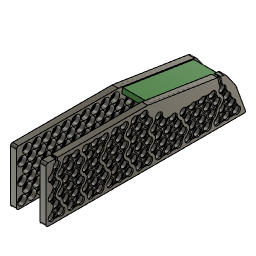
battery v13 (Autodesk Fusion 360 design; units mm, degrees)
Autodesk Fusion 360 part; units mm, degrees
note: some values were not read from the file. Set by a fixed rule: which face or edge a step refers to.
(part 1 of 2)
sketch "Sketch1" plane through (0, 0, 0) normal (1, 0, 0) x (0, 1, 0)
  circle A0 centre (0, 0) radius 9.25
  circle A1 centre (19.5, 0) radius 9.25
  circle A2 centre (39, 0) radius 9.25
  circle A3 centre (58.5, 0) radius 9.25
  circle A4 centre (78, 0) radius 9.25
  circle A5 centre (97.5, 0) radius 9.25
  circle A6 centre (117, 0) radius 9.25
  circle A7 centre (136.5, 0) radius 9.25
  circle A8 centre (156, 0) radius 9.25
  circle A9 centre (175.5, 0) radius 9.25
  circle A10 centre (195, 0) radius 9.25
  circle A11 centre (214.5, 0) radius 9.25
  circle A12 centre (234, 0) radius 9.25
  circle A13 centre (253.5, 0) radius 9.25
  circle A14 centre (273, 0) radius 9.25
  circle A15 centre (292.5, 0) radius 9.25
  circle A16 centre (312, 0) radius 9.25
  circle A17 centre (331.5, 0) radius 9.25
  circle A18 centre (351, 0) radius 9.25
  circle A19 centre (127, 17) radius 9.25
  circle A20 centre (88, 17) radius 9.25
  circle A21 centre (283, 17) radius 9.25
  circle A22 centre (263.5, 17) radius 9.25
  circle A23 centre (10, 17) radius 9.25
  circle A24 centre (68.5, 17) radius 9.25
  circle A25 centre (185.5, 17) radius 9.25
  circle A26 centre (205, 17) radius 9.25
  circle A27 centre (107.5, 17) radius 9.25
  circle A28 centre (166, 17) radius 9.25
  circle A29 centre (-9.5, 17) radius 9.25
  circle A30 centre (302.5, 17) radius 9.25
  circle A31 centre (146.5, 17) radius 9.25
  circle A32 centre (224.5, 17) radius 9.25
  circle A33 centre (49, 17) radius 9.25
  circle A34 centre (341.5, 17) radius 9.25
  circle A35 centre (322, 17) radius 9.25
  circle A36 centre (244, 17) radius 9.25
  circle A37 centre (29.5, 17) radius 9.25
  circle A38 centre (58.5, 34) radius 9.25
  circle A39 centre (214.5, 34) radius 9.25
  circle A40 centre (136.5, 34) radius 9.25
  circle A41 centre (19.5, 34) radius 9.25
  circle A42 centre (195, 34) radius 9.25
  circle A43 centre (78, 34) radius 9.25
  circle A44 centre (175.5, 34) radius 9.25
  circle A45 centre (253.5, 34) radius 9.25
  circle A46 centre (331.5, 34) radius 9.25
  circle A47 centre (0, 34) radius 9.25
  circle A48 centre (234, 34) radius 9.25
  circle A49 centre (39, 34) radius 9.25
  circle A50 centre (156, 34) radius 9.25
  circle A51 centre (97.5, 34) radius 9.25
  circle A52 centre (117, 34) radius 9.25
  circle A53 centre (292.5, 34) radius 9.25
  circle A54 centre (312, 34) radius 9.25
  circle A55 centre (273, 34) radius 9.25
  circle A56 centre (185.4697, 51) radius 9.25
  circle A57 centre (263.4697, 51) radius 9.25
  circle A58 centre (321.9697, 51) radius 9.25
  circle A59 centre (224.4697, 51) radius 9.25
  circle A60 centre (9.9697, 51) radius 9.25
  circle A61 centre (243.9697, 51) radius 9.25
  circle A62 centre (282.9697, 51) radius 9.25
  circle A63 centre (302.4697, 51) radius 9.25
  circle A64 centre (48.9697, 51) radius 9.25
  circle A65 centre (29.4697, 51) radius 9.25
  circle A66 centre (-9.5303, 51) radius 9.25
  circle A67 centre (107.4697, 51) radius 9.25
  circle A68 centre (165.9697, 51) radius 9.25
  circle A69 centre (204.9697, 51) radius 9.25
  circle A70 centre (87.9697, 51) radius 9.25
  circle A71 centre (68.4697, 51) radius 9.25
  circle A72 centre (146.4697, 51) radius 9.25
  circle A73 centre (126.9697, 51) radius 9.25
  circle A74 centre (-19.5, 34) radius 9.25
  circle A75 centre (-19.5, 0) radius 9.25
  circle A76 centre (351, 0) radius 7
  circle A77 centre (331.5, 0) radius 7
  circle A78 centre (312, 0) radius 7
  circle A79 centre (292.5, 0) radius 7
  circle A80 centre (273, 0) radius 7
  circle A81 centre (253.5, 0) radius 7
  circle A82 centre (234, 0) radius 7
  circle A83 centre (214.5, 0) radius 7
  circle A84 centre (195, 0) radius 7
  circle A85 centre (175.5, 0) radius 7
  circle A86 centre (156, 0) radius 7
  circle A87 centre (136.5, 0) radius 7
  circle A88 centre (117, 0) radius 7
  circle A89 centre (97.5, 0) radius 7
  circle A90 centre (78, 0) radius 7
  circle A91 centre (58.5, 0) radius 7
  circle A92 centre (39, 0) radius 7
  circle A93 centre (19.5, 0) radius 7
  circle A94 centre (0, 0) radius 7
  circle A95 centre (-19.5, 0) radius 7
  circle A96 centre (341.5, 17) radius 7
  circle A97 centre (331.5, 34) radius 7
  circle A98 centre (321.9697, 51) radius 7
  circle A99 centre (322, 17) radius 7
  circle A100 centre (312, 34) radius 7
  circle A101 centre (302.4697, 51) radius 7
  circle A102 centre (302.5, 17) radius 7
  circle A103 centre (292.5, 34) radius 7
  circle A104 centre (282.9697, 51) radius 7
  circle A105 centre (283, 17) radius 7
  circle A106 centre (273, 34) radius 7
  circle A107 centre (263.4697, 51) radius 7
  circle A108 centre (263.5, 17) radius 7
  circle A109 centre (253.5, 34) radius 7
  circle A110 centre (243.9697, 51) radius 7
  circle A111 centre (244, 17) radius 7
  circle A112 centre (234, 34) radius 7
  circle A113 centre (224.4697, 51) radius 7
  circle A114 centre (224.5, 17) radius 7
  circle A115 centre (214.5, 34) radius 7
  circle A116 centre (204.9697, 51) radius 7
  circle A117 centre (205, 17) radius 7
  circle A118 centre (195, 34) radius 7
  circle A119 centre (185.4697, 51) radius 7
  circle A120 centre (185.5, 17) radius 7
  circle A121 centre (175.5, 34) radius 7
  circle A122 centre (165.9697, 51) radius 7
  circle A123 centre (166, 17) radius 7
  circle A124 centre (156, 34) radius 7
  circle A125 centre (146.4697, 51) radius 7
  circle A126 centre (146.5, 17) radius 7
  circle A127 centre (136.5, 34) radius 7
  circle A128 centre (126.9697, 51) radius 7
  circle A129 centre (127, 17) radius 7
  circle A130 centre (117, 34) radius 7
  circle A131 centre (107.4697, 51) radius 7
  circle A132 centre (107.5, 17) radius 7
  circle A133 centre (97.5, 34) radius 7
  circle A134 centre (87.9697, 51) radius 7
  circle A135 centre (88, 17) radius 7
  circle A136 centre (78, 34) radius 7
  circle A137 centre (68.4697, 51) radius 7
  circle A138 centre (68.5, 17) radius 7
  circle A139 centre (58.5, 34) radius 7
  circle A140 centre (48.9697, 51) radius 7
  circle A141 centre (49, 17) radius 7
  circle A142 centre (39, 34) radius 7
  circle A143 centre (29.4697, 51) radius 7
  circle A144 centre (29.5, 17) radius 7
  circle A145 centre (19.5, 34) radius 7
  circle A146 centre (9.9697, 51) radius 7
  circle A147 centre (10, 17) radius 7
  circle A148 centre (0, 34) radius 7
  circle A149 centre (-9.5303, 51) radius 7
  circle A150 centre (-9.5, 17) radius 7
  circle A151 centre (-19.5, 34) radius 7
  line L0 (-31, -12) -> (-31, 98)
  line L1 (-31, -12) -> (369, -12)
  line L2 (-31, 98) -> (172.6327, 98)
  line L3 (327.7275, 73.6318) -> (348.4062, 44.7862)
  line L4 (348.4062, 44.7862) -> (369, -12)
  line L5 (172.6327, 98) -> (327.7275, 73.6318)
  circle A152 centre (-19.5, 68) radius 9.25
  circle A153 centre (-19.5, 68) radius 7
  circle A154 centre (-9.5303, 85) radius 9.25
  circle A155 centre (-9.5303, 85) radius 7
  circle A156 centre (0, 68) radius 9.25
  circle A157 centre (0, 68) radius 7
  circle A158 centre (9.9697, 85) radius 9.25
  circle A159 centre (9.9697, 85) radius 7
  circle A160 centre (19.5, 68) radius 9.25
  circle A161 centre (19.5, 68) radius 7
  circle A162 centre (29.4697, 85) radius 9.25
  circle A163 centre (29.4697, 85) radius 7
  circle A164 centre (39, 68) radius 9.25
  circle A165 centre (39, 68) radius 7
  circle A166 centre (48.9697, 85) radius 9.25
  circle A167 centre (48.9697, 85) radius 7
  circle A168 centre (58.5, 68) radius 9.25
  circle A169 centre (58.5, 68) radius 7
  circle A170 centre (68.4697, 85) radius 9.25
  circle A171 centre (68.4697, 85) radius 7
  circle A172 centre (78, 68) radius 9.25
  circle A173 centre (78, 68) radius 7
  circle A174 centre (87.9697, 85) radius 9.25
  circle A175 centre (87.9697, 85) radius 7
  circle A176 centre (97.5, 68) radius 9.25
  circle A177 centre (97.5, 68) radius 7
  circle A178 centre (107.4697, 85) radius 9.25
  circle A179 centre (107.4697, 85) radius 7
  circle A180 centre (117, 68) radius 9.25
  circle A181 centre (117, 68) radius 7
  circle A182 centre (126.9697, 85) radius 9.25
  circle A183 centre (126.9697, 85) radius 7
  circle A184 centre (136.5, 68) radius 9.25
  circle A185 centre (136.5, 68) radius 7
  circle A186 centre (146.4697, 85) radius 9.25
  circle A187 centre (146.4697, 85) radius 7
  circle A188 centre (156, 68) radius 9.25
  circle A189 centre (156, 68) radius 7
  circle A190 centre (165.9697, 85) radius 9.25
  circle A191 centre (165.9697, 85) radius 7
  circle A192 centre (175.5, 68) radius 9.25
  circle A193 centre (175.5, 68) radius 7
  circle A194 centre (195, 68) radius 7
  circle A195 centre (195, 68) radius 9.25
  point P0 (-9.5, 17)
  point P1 (0, 34)
  point P2 (-9.5303, 51)
  dimension "d4" = 19.5
  dimension "d5" = 0
  dimension "d8" = 19.5
  dimension "d9" = 0
  dimension "d13" = 19.5
  dimension "d14" = 0
  dimension "d18" = 19.5
  dimension "d19" = 0
  dimension "d28" = 14
  dimension "d31" = -19.5
  dimension "d32" = 0
  dimension "d33" = 14
  dimension "d34" = 14
  dimension "d35" = 14
  dimension "d40" = -19.5
  dimension "d41" = 0
  dimension "d48" = 12
  dimension "d252" = 18.5
  dimension "d253" = 18.5
  dimension "d254" = 17
  dimension "d255" = 17
  dimension "d256" = 18.5
  dimension "d257" = 19.5
  dimension "d258" = 18.5
  dimension "d259" = 18.5
  dimension "d260" = 17
  dimension "d262" = 18.5
  dimension "d265" = 17
  dimension "d268" = 400
  dimension "d271" = 19.5
  dimension "d272" = 34
  dimension "d273" = 110
  dimension "d276" = 19.5
  dimension "d277" = 19.5
  constraint coincident A0.centre A94.centre
  constraint coincident P0 A29.centre
  constraint coincident P1 A47.centre
  constraint coincident P2 A66.centre
  constraint concentric A18 A76
  constraint concentric A34 A96
  constraint concentric A46 A97
  constraint concentric A58 A98
  constraint vertical L0
  constraint horizontal L1
  constraint horizontal L2
  constraint coincident A75.centre A95.centre
  constraint coincident A74.centre A151.centre
  measures "d28" diameter of A76
  measures "d33" diameter of A96
  measures "d34" diameter of A97
  measures "d35" diameter of A98
  measures "d48" distance of A75.centre L1
  measures "d252" diameter of A0
  measures "d253" diameter of A34
  measures "d254" vertical distance of A18.centre A34.centre
  measures "d255" vertical distance of A46.centre A34.centre
  measures "d256" diameter of A75
  measures "d257" horizontal distance of P1 A74.centre
  measures "d258" diameter of A74
  measures "d259" diameter of A47
  measures "d260" vertical distance of P1 P2
  measures "d262" diameter of A58
  measures "d265" vertical distance of P0 A74.centre
  measures "d268" distance of L0.start L1.end
  measures "d273" distance of L0.end L0.start
extrude "Extrude1" add sketch "Sketch1" along normal blind 12 contours L0 L1 L2 L3 L4 L5 makes body 1
extrude "Extrude2" add sketch "Sketch1" along normal blind 3 contours A0 | A1 | A2 | A3 | A4 | A5 | A6 | A7 | A8 | A9 | A10 | A11 | A12 | A13 | A14 | A15 | A16 | A17 | A18 | A19 | A20 | A21 | A22 | A23 | A24 | A25 | A26 | A27 | A28 | A29 | A30 | A31 | A32 | A33 | A34 | A35 | A36 | A37 | A38 | A39 | A40 | A41 | A42 | A43 | A44 | A45 | A46 | A47 | A48 | A49 | A50 | A51 | A52 | A53 | A54 | A55 | A56 | A57 | A58 | A59 | A60 | A61 | A62 | A63 | A64 | A65 | A66 | A67 | A68 | A69 | A70 | A71 | A72 | A73 | A74 | A75 | A152 | A154 | A156 | A158 | A160 | A162 | A164 | A166 | A168 | A170 | A172 | A174 | A176 | A178 | A180 | A182 | A184 | A186 | A188 | A190 | A192 | A195 bodies 1
sketch "Sketch2" plane through (0, 0, 0) normal (-1, 0, 0) x (0, -1, 0)
  circle A0 centre (-331.5, 0) radius 7 construction
  circle A1 centre (-322, 17) radius 7 construction
  circle A2 centre (-312, 34) radius 7 construction
  circle A3 centre (-283, 17) radius 7 construction
  circle A4 centre (-273, 34) radius 7 construction
  circle A5 centre (-244, 17) radius 7 construction
  circle A6 centre (-224.5, 17) radius 7 construction
  circle A7 centre (-214.5, 34) radius 7 construction
  circle A8 centre (-185.5, 17) radius 7 construction
  circle A9 centre (-117, 0) radius 7 construction
  circle A10 centre (-146.5, 17) radius 7 construction
  circle A11 centre (-165.9697, 51) radius 7 construction
  circle A12 centre (-117, 34) radius 7 construction
  circle A13 centre (-88, 17) radius 7 construction
  circle A14 centre (-68.5, 17) radius 7 construction
  circle A15 centre (-39, 34) radius 7 construction
  circle A16 centre (-29.4697, 51) radius 7 construction
  circle A17 centre (-9.9697, 51) radius 7 construction
  circle A18 centre (0, 0) radius 7 construction
  circle A19 centre (9.5, 17) radius 7 construction
  circle A20 centre (19.5, 34) radius 7 construction
  circle A21 centre (9.5303, 51) radius 7 construction
  circle A22 centre (-19.5, 0) radius 7 construction
  circle A23 centre (-49, 17) radius 7 construction
  circle A24 centre (-78, 34) radius 7 construction
  circle A25 centre (-78, 0) radius 7 construction
  circle A26 centre (-126.9697, 51) radius 7 construction
  circle A27 centre (-185.4697, 51) radius 7 construction
  circle A28 centre (-136.5, 34) radius 7 construction
  circle A29 centre (-156, 0) radius 7 construction
  circle A30 centre (-195, 34) radius 7 construction
  circle A31 centre (-205, 17) radius 7 construction
  circle A32 centre (-234, 34) radius 7 construction
  circle A33 centre (-253.5, 34) radius 7 construction
  circle A34 centre (-263.5, 17) radius 7 construction
  circle A35 centre (-292.5, 34) radius 7 construction
  circle A36 centre (-302.5, 17) radius 7 construction
  circle A37 centre (-331.5, 34) radius 7 construction
  circle A38 centre (-351, 0) radius 7 construction
  circle A39 centre (-312, 0) radius 7 construction
  circle A40 centre (-321.9697, 51) radius 7 construction
  circle A41 centre (-273, 0) radius 7 construction
  circle A42 centre (-282.9697, 51) radius 7 construction
  circle A43 centre (-234, 0) radius 7 construction
  circle A44 centre (-214.5, 0) radius 7 construction
  circle A45 centre (-224.4697, 51) radius 7 construction
  circle A46 centre (-175.5, 0) radius 7 construction
  circle A47 centre (-136.5, 0) radius 7 construction
  circle A48 centre (-156, 34) radius 7 construction
  circle A49 centre (-146.4697, 51) radius 7 construction
  circle A50 centre (-107.5, 17) radius 7 construction
  circle A51 centre (-97.5, 34) radius 7 construction
  circle A52 centre (-58.5, 0) radius 7 construction
  circle A53 centre (-58.5, 34) radius 7 construction
  circle A54 centre (-19.5, 34) radius 7 construction
  circle A55 centre (-10, 17) radius 7 construction
  circle A56 centre (19.5, 0) radius 7 construction
  circle A57 centre (0, 34) radius 7 construction
  circle A58 centre (-29.5, 17) radius 7 construction
  circle A59 centre (-48.9697, 51) radius 7 construction
  circle A60 centre (-39, 0) radius 7 construction
  circle A61 centre (-68.4697, 51) radius 7 construction
  circle A62 centre (-87.9697, 51) radius 7 construction
  circle A63 centre (-97.5, 0) radius 7 construction
  circle A64 centre (-107.4697, 51) radius 7 construction
  circle A65 centre (-175.5, 34) radius 7 construction
  circle A66 centre (-127, 17) radius 7 construction
  circle A67 centre (-166, 17) radius 7 construction
  circle A68 centre (-204.9697, 51) radius 7 construction
  circle A69 centre (-195, 0) radius 7 construction
  circle A70 centre (-243.9697, 51) radius 7 construction
  circle A71 centre (-263.4697, 51) radius 7 construction
  circle A72 centre (-253.5, 0) radius 7 construction
  circle A73 centre (-302.4697, 51) radius 7 construction
  circle A74 centre (-292.5, 0) radius 7 construction
  circle A75 centre (-341.5, 17) radius 7 construction
  line L0 (-327.7275, 73.6318) -> (-348.4062, 44.7862) construction
  line L1 (-348.4062, 44.7862) -> (-369, -12) construction
  line L2 (-369, -12) -> (31, -12)
  line L3 (31, -12) -> (31, 98)
  line L4 (31, 98) -> (-172.6327, 98)
  line L5 (9.5303, 85) -> (19.4283, 67.8265) construction
  line L6 (19.4283, 67.8265) -> (9.5303, 51) construction
  line L7 (9.5303, 51) -> (19.5, 34) construction
  line L8 (19.5, 34) -> (9.5, 17) construction
  line L9 (0, 0) -> (9.5, 17) construction
  line L10 (-19.5, 0) -> (-10, 17) construction
  line L11 (-10, 17) -> (0, 34) construction
  line L12 (0, 34) -> (-9.9697, 51) construction
  line L13 (-9.9697, 51) -> (0, 68) construction
  line L14 (0, 68) -> (-9.9697, 85) construction
  line L15 (-9.9697, 85) -> (-19.5, 68) construction
  line L16 (-19.5, 68) -> (-9.9697, 51) construction
  line L17 (-39, 0) -> (-29.5, 17) construction
  line L18 (-29.5, 17) -> (-19.5, 34) construction
  line L19 (-19.5, 34) -> (-29.4697, 51) construction
  line L20 (-29.4697, 51) -> (-39, 68) construction
  line L21 (-39, 68) -> (-29.4697, 85) construction
  line L22 (-39, 34) -> (-29.5, 17) construction
  line L23 (-39, 34) -> (-29.4697, 51) construction
  line L24 (-58.5, 0) -> (-49, 17) construction
  line L25 (-49, 17) -> (-58.5, 34) construction
  line L26 (-58.5, 34) -> (-48.9697, 51) construction
  line L27 (-48.9697, 51) -> (-58.5, 68) construction
  line L28 (-58.5, 68) -> (-48.9697, 85) construction
  line L29 (-48.9697, 85) -> (-68.4697, 85) construction
  line L30 (-68.4697, 85) -> (-58.5, 68) construction
  line L31 (-78, 0) -> (-68.5, 17) construction
  line L32 (-68.5, 17) -> (-78, 34) construction
  line L33 (-78, 34) -> (-68.4697, 51) construction
  line L34 (-68.4697, 51) -> (-76.7499, 65.5682) construction
  line L35 (-76.7499, 65.5682) -> (-87.9697, 85) construction
  line L36 (-78, 0) -> (-88, 17) construction
  line L37 (-88, 17) -> (-78, 34) construction
  line L38 (-97.5, 0) -> (-107.5, 17) construction
  line L39 (-107.5, 17) -> (-97.5, 34) construction
  line L40 (-97.5, 34) -> (-87.9697, 51) construction
  line L41 (-87.9697, 51) -> (-97.5, 68) construction
  line L42 (-97.5, 68) -> (-107.4697, 51) construction
  line L43 (-107.4697, 51) -> (-97.5, 34) construction
  line L44 (-97.5, 68) -> (-107.4697, 85) construction
  line L45 (-126.9697, 85) -> (-117, 68) construction
  line L46 (-117, 68) -> (-126.9697, 51) construction
  line L47 (-126.9697, 51) -> (-117, 34) construction
  line L48 (-117, 34) -> (-127, 17) construction
  line L49 (-127, 17) -> (-117, 0) construction
  line L50 (-117, 0) -> (-136.5, 0) construction
  line L51 (-136.5, 0) -> (-127, 17) construction
  line L52 (-156, 0) -> (-146.5, 17) construction
  line L53 (-146.5, 17) -> (-136.5, 34) construction
  line L54 (-136.5, 34) -> (-146.4697, 51) construction
  line L55 (-146.4697, 51) -> (-136.5, 68) construction
  line L56 (-136.5, 68) -> (-146.4697, 85) construction
  line L57 (-156, 34) -> (-146.5, 17) construction
  line L58 (-156, 34) -> (-146.4697, 51) construction
  line L59 (-165.9697, 85) -> (-156, 68) construction
  line L60 (-175.5, 68) -> (-165.9697, 85) construction
  line L61 (-165.9697, 51) -> (-156, 68) construction
  line L62 (-165.9697, 51) -> (-175.5, 34) construction
  line L63 (-175.5, 34) -> (-166, 17) construction
  line L64 (-166, 17) -> (-175.5, 0) construction
  line L65 (-175.5, 68) -> (-165.9697, 51) construction
  line L66 (-195, 0) -> (-185.5, 17) construction
  line L67 (-185.5, 17) -> (-195, 34) construction
  line L68 (-195, 34) -> (-185.4697, 51) construction
  line L69 (-185.4697, 51) -> (-195, 68) construction
  line L70 (-204.9697, 51) -> (-195, 34) construction
  line L71 (-195, 68) -> (-204.9697, 51) construction
  line L72 (-205, 17) -> (-195, 0) construction
  line L73 (-205, 17) -> (-195, 34) construction
  line L74 (-214.5, 34) -> (-224.4697, 51) construction
  line L75 (-224.4697, 51) -> (-234, 34) construction
  line L76 (-224.5, 17) -> (-214.5, 0) construction
  line L77 (-214.5, 0) -> (-234, 0) construction
  line L78 (-224.5, 17) -> (-214.5, 34) construction
  line L79 (-234, 0) -> (-244, 17) construction
  line L80 (-244, 17) -> (-234, 34) construction
  line L81 (-243.9697, 51) -> (-263.4697, 51) construction
  line L82 (-253.5, 34) -> (-243.9697, 51) construction
  line L83 (-253.5, 34) -> (-263.5, 17) construction
  line L84 (-263.5, 17) -> (-253.5, 0) construction
  line L85 (-253.5, 0) -> (-273, 0) construction
  line L86 (-273, 0) -> (-263.5, 17) construction
  line L87 (-263.5, 17) -> (-273, 34) construction
  line L88 (-273, 34) -> (-263.4697, 51) construction
  line L89 (-282.9697, 51) -> (-292.5, 34) construction
  line L90 (-292.5, 34) -> (-283, 17) construction
  line L91 (-283, 17) -> (-292.5, 0) construction
  line L92 (-292.5, 0) -> (-302.5, 17) construction
  line L93 (-302.5, 17) -> (-312, 34) construction
  line L94 (-312, 34) -> (-302.4697, 51) construction
  line L95 (-351, 0) -> (-341.5, 17) construction
  line L96 (-341.5, 17) -> (-331.5, 34) construction
  line L97 (-331.5, 34) -> (-322, 17) construction
  line L98 (-351, 0) -> (-331.5, 0) construction
  line L99 (-312, 0) -> (-322, 17) construction
  line L100 (-331.5, 0) -> (-312, 0) construction
  line L101 (-321.9697, 51) -> (-331.5, 34) construction
  line L102 (-302.4697, 51) -> (-282.9697, 51) construction
  line L103 (-172.6327, 98) -> (-327.7275, 73.6318) construction
  circle A76 centre (-175.5, 68) radius 7 construction
  circle A77 centre (-146.4697, 85) radius 7 construction
  circle A78 centre (-107.4697, 85) radius 7 construction
  circle A79 centre (-68.4697, 85) radius 7 construction
  circle A80 centre (-29.4697, 85) radius 7 construction
  circle A81 centre (9.5303, 85) radius 7 construction
  circle A82 centre (-9.9697, 85) radius 7 construction
  circle A83 centre (-39, 68) radius 7 construction
  circle A84 centre (-78, 68) radius 7 construction
  circle A85 centre (-126.9697, 85) radius 7 construction
  circle A86 centre (-156, 68) radius 7 construction
  circle A87 centre (-136.5, 68) radius 7 construction
  circle A88 centre (-97.5, 68) radius 7 construction
  circle A89 centre (-58.5, 68) radius 7 construction
  circle A90 centre (-19.5, 68) radius 7 construction
  circle A91 centre (19.5, 68) radius 7 construction
  circle A92 centre (0, 68) radius 7 construction
  circle A93 centre (-48.9697, 85) radius 7 construction
  circle A94 centre (-87.9697, 85) radius 7 construction
  circle A95 centre (-117, 68) radius 7 construction
  circle A96 centre (-165.9697, 85) radius 7 construction
  circle A97 centre (-195, 68) radius 7 construction
  line L104 (-58.5977, 78.0505) -> (-57.5048, 80) construction
  line L105 (-57.5048, 80) -> (-59.741, 80) construction
  line L106 (-59.741, 80) -> (-58.5977, 78.0505) construction
  line L107 (-331.5, 0) -> (-322, 17) construction
  line L108 (-341.5, 17) -> (-331.5, 0) construction
  line L109 (-322, 17) -> (-341.5, 17) construction
  line L110 (-302.5, 17) -> (-283, 17) construction
  line L111 (-292.5, 34) -> (-312, 34) construction
  line L112 (-292.5, 34) -> (-302.5, 17) construction
  line L113 (-292.5, 34) -> (-302.4697, 51) construction
  line L114 (-253.5, 34) -> (-263.4697, 51) construction
  line L115 (-273, 34) -> (-253.5, 34) construction
  line L116 (-244, 17) -> (-224.5, 17) construction
  line L117 (-234, 0) -> (-224.5, 17) construction
  line L118 (-224.5, 17) -> (-234, 34) construction
  line L119 (-214.5, 34) -> (-234, 34) construction
  line L120 (-185.5, 17) -> (-205, 17) construction
  line L121 (-185.4697, 51) -> (-204.9697, 51) construction
  line L122 (-175.5, 68) -> (-156, 68) construction
  line L123 (-156, 34) -> (-136.5, 34) construction
  line L124 (-107.4697, 51) -> (-87.9697, 51) construction
  line L125 (-88, 17) -> (-68.5, 17) construction
  line L126 (-39, 34) -> (-19.5, 34) construction
  line L127 (-19.5, 68) -> (0, 68) construction
  line L128 (19.5, 0) -> (9.5, 17) construction
  line L129 (0, 0) -> (19.5, 0) construction
  line L130 (-335.5965, 16.8256) -> (-329.3321, 6.1762)
  line L131 (-344.2941, 12) -> (-344.3597, 12)
  line L132 (-344.3597, 12) -> (-337.7357, 0.7392)
  line L133 (-335.5965, 16.8256) -> (-337.4264, 19.9364)
  line L134 (-344.3597, 12) -> (-346.7144, 16.0029)
  line L135 (-337.7357, 0.7392) -> (-335.7099, -2.7047)
  line L136 (-329.3321, 6.1762) -> (-326.75, 1.781)
  line L137 (-335.7099, -2.7047) -> (-326.75, 1.781)
  line L138 (-337.4264, 19.9364) -> (-346.7144, 16.0029)
  line L139 (5.1983, 82.5033) -> (15.0963, 65.3298)
  line L140 (13.8623, 87.4967) -> (23.7603, 70.3233)
  line L141 (23.7603, 70.3233) -> (74.0347, -16.9057)
  line L142 (15.0963, 65.3298) -> (63.6851, -18.9746)
  line L143 (15.1903, 36.5351) -> (5.1903, 19.5351)
  line L144 (23.8097, 31.4649) -> (13.8097, 14.4649)
  line L145 (23.8097, 31.4649) -> (58.8391, 91.015)
  line L146 (15.1903, 36.5351) -> (49.1846, 94.3253)
  line L147 (5.1903, 19.5351) -> (-25, -30)
  line L148 (13.8097, 14.4649) -> (-15, -35)
  line L149 (5.1983, 82.5033) -> (0.3906, 90.845)
  line L150 (-5.6377, 87.4967) -> (4.2603, 70.3233)
  line L151 (4.2603, 70.3233) -> (54.5347, -16.9057)
  line L152 (-14.3017, 82.5033) -> (-19.1094, 90.845)
  line L153 (-14.3017, 82.5033) -> (-4.4037, 65.3298)
  line L154 (-4.4037, 65.3298) -> (44.1851, -18.9746)
  line L155 (-25.1377, 87.4967) -> (-15.2397, 70.3233)
  line L156 (-15.2397, 70.3233) -> (35.0347, -16.9057)
  line L157 (-33.8017, 82.5033) -> (-38.6094, 90.845)
  line L158 (-33.8017, 82.5033) -> (-23.9037, 65.3298)
  line L159 (-23.9037, 65.3298) -> (24.6851, -18.9746)
  line L160 (-44.6377, 87.4967) -> (-34.7397, 70.3233)
  line L161 (-34.7397, 70.3233) -> (15.5347, -16.9057)
  line L162 (-53.3017, 82.5033) -> (-58.1094, 90.845)
  line L163 (-53.3017, 82.5033) -> (-43.4037, 65.3298)
  line L164 (-43.4037, 65.3298) -> (5.1851, -18.9746)
  line L165 (-64.1377, 87.4967) -> (-54.2397, 70.3233)
  line L166 (-54.2397, 70.3233) -> (-3.9653, -16.9057)
  line L167 (-72.8017, 82.5033) -> (-77.6094, 90.845)
  line L168 (-72.8017, 82.5033) -> (-62.9037, 65.3298)
  line L169 (-62.9037, 65.3298) -> (-14.3149, -18.9746)
  line L170 (-83.6377, 87.4967) -> (-73.7397, 70.3233)
  line L171 (-73.7397, 70.3233) -> (-23.4653, -16.9057)
  line L172 (-92.3017, 82.5033) -> (-97.1094, 90.845)
  line L173 (-92.3017, 82.5033) -> (-82.4037, 65.3298)
  line L174 (-82.4037, 65.3298) -> (-33.8149, -18.9746)
  line L175 (-103.1377, 87.4967) -> (-93.2397, 70.3233)
  line L176 (-93.2397, 70.3233) -> (-42.9653, -16.9057)
  line L177 (-111.8017, 82.5033) -> (-116.6094, 90.845)
  line L178 (-111.8017, 82.5033) -> (-101.9037, 65.3298)
  line L179 (-101.9037, 65.3298) -> (-53.3149, -18.9746)
  line L180 (-122.6377, 87.4967) -> (-112.7397, 70.3233)
  line L181 (-112.7397, 70.3233) -> (-62.4653, -16.9057)
  line L182 (-131.3017, 82.5033) -> (-136.1094, 90.845)
  line L183 (-131.3017, 82.5033) -> (-121.4037, 65.3298)
  line L184 (-121.4037, 65.3298) -> (-72.8149, -18.9746)
  line L185 (-142.1377, 87.4967) -> (-132.2397, 70.3233)
  line L186 (-132.2397, 70.3233) -> (-81.9653, -16.9057)
  line L187 (-150.8017, 82.5033) -> (-155.6094, 90.845)
  line L188 (-150.8017, 82.5033) -> (-140.9037, 65.3298)
  line L189 (-140.9037, 65.3298) -> (-92.3149, -18.9746)
  line L190 (-161.6377, 87.4967) -> (-151.7397, 70.3233)
  line L191 (-151.7397, 70.3233) -> (-101.4653, -16.9057)
  line L192 (-170.3017, 82.5033) -> (-175.1094, 90.845)
  line L193 (-170.3017, 82.5033) -> (-160.4037, 65.3298)
  line L194 (-160.4037, 65.3298) -> (-111.8149, -18.9746)
  line L195 (-181.1377, 87.4967) -> (-171.2397, 70.3233)
  line L196 (-171.2397, 70.3233) -> (-120.9653, -16.9057)
  line L197 (-189.8017, 82.5033) -> (-194.6094, 90.845)
  line L198 (-189.8017, 82.5033) -> (-179.9037, 65.3298)
  line L199 (-179.9037, 65.3298) -> (-131.3149, -18.9746)
  line L200 (-200.6377, 87.4967) -> (-190.7397, 70.3233)
  line L201 (-190.7397, 70.3233) -> (-140.4653, -16.9057)
  line L202 (-209.3017, 82.5033) -> (-214.1094, 90.845)
  line L203 (-209.3017, 82.5033) -> (-199.4037, 65.3298)
  line L204 (-199.4037, 65.3298) -> (-150.8149, -18.9746)
  line L205 (-220.1377, 87.4967) -> (-210.2397, 70.3233)
  line L206 (-210.2397, 70.3233) -> (-159.9653, -16.9057)
  line L207 (-228.8017, 82.5033) -> (-233.6094, 90.845)
  line L208 (-228.8017, 82.5033) -> (-218.9037, 65.3298)
  line L209 (-218.9037, 65.3298) -> (-170.3149, -18.9746)
  line L210 (-239.6377, 87.4967) -> (-229.7397, 70.3233)
  line L211 (-229.7397, 70.3233) -> (-179.4653, -16.9057)
  line L212 (-248.3017, 82.5033) -> (-253.1094, 90.845)
  line L213 (-248.3017, 82.5033) -> (-238.4037, 65.3298)
  line L214 (-238.4037, 65.3298) -> (-189.8149, -18.9746)
  line L215 (-259.1377, 87.4967) -> (-249.2397, 70.3233)
  line L216 (-249.2397, 70.3233) -> (-198.9653, -16.9057)
  line L217 (-267.8017, 82.5033) -> (-272.6094, 90.845)
  line L218 (-267.8017, 82.5033) -> (-257.9037, 65.3298)
  line L219 (-257.9037, 65.3298) -> (-209.3149, -18.9746)
  line L220 (-278.6377, 87.4967) -> (-268.7397, 70.3233)
  line L221 (-268.7397, 70.3233) -> (-218.4653, -16.9057)
  line L222 (-287.3017, 82.5033) -> (-292.1094, 90.845)
  line L223 (-287.3017, 82.5033) -> (-277.4037, 65.3298)
  line L224 (-277.4037, 65.3298) -> (-228.8149, -18.9746)
  line L225 (-298.1377, 87.4967) -> (-288.2397, 70.3233)
  line L226 (-288.2397, 70.3233) -> (-237.9653, -16.9057)
  line L227 (-306.8017, 82.5033) -> (-311.6094, 90.845)
  line L228 (-306.8017, 82.5033) -> (-296.9037, 65.3298)
  line L229 (-296.9037, 65.3298) -> (-248.3149, -18.9746)
  line L230 (-317.6377, 87.4967) -> (-307.7397, 70.3233)
  line L231 (-307.7397, 70.3233) -> (-257.4653, -16.9057)
  line L232 (-326.3017, 82.5033) -> (-331.1094, 90.845)
  line L233 (-326.3017, 82.5033) -> (-316.4037, 65.3298)
  line L234 (-316.4037, 65.3298) -> (-267.8149, -18.9746)
  line L235 (-337.1377, 87.4967) -> (-327.2397, 70.3233)
  line L236 (-327.2397, 70.3233) -> (-276.9653, -16.9057)
  line L237 (-345.8017, 82.5033) -> (-350.6094, 90.845)
  line L238 (-345.8017, 82.5033) -> (-335.9037, 65.3298)
  line L239 (-335.9037, 65.3298) -> (-287.3149, -18.9746)
  line L240 (-356.6377, 87.4967) -> (-346.7397, 70.3233)
  line L241 (-346.7397, 70.3233) -> (-296.4653, -16.9057)
  line L242 (-365.3017, 82.5033) -> (-370.1094, 90.845)
  line L243 (-365.3017, 82.5033) -> (-355.4037, 65.3298)
  line L244 (-355.4037, 65.3298) -> (-306.8149, -18.9746)
  line L245 (-5.6903, 14.4649) -> (-34.5, -35)
  line L246 (4.3097, 31.4649) -> (-5.6903, 14.4649)
  line L247 (4.3097, 31.4649) -> (39.3391, 91.015)
  line L248 (-14.3097, 19.5351) -> (-44.5, -30)
  line L249 (-4.3097, 36.5351) -> (-14.3097, 19.5351)
  line L250 (-4.3097, 36.5351) -> (29.6846, 94.3253)
  line L251 (-25.1903, 14.4649) -> (-54, -35)
  line L252 (-15.1903, 31.4649) -> (-25.1903, 14.4649)
  line L253 (-15.1903, 31.4649) -> (19.8391, 91.015)
  line L254 (-33.8097, 19.5351) -> (-64, -30)
  line L255 (-23.8097, 36.5351) -> (-33.8097, 19.5351)
  line L256 (-23.8097, 36.5351) -> (10.1846, 94.3253)
  line L257 (-44.6903, 14.4649) -> (-73.5, -35)
  line L258 (-34.6903, 31.4649) -> (-44.6903, 14.4649)
  line L259 (-34.6903, 31.4649) -> (0.3391, 91.015)
  line L260 (-53.3097, 19.5351) -> (-83.5, -30)
  line L261 (-43.3097, 36.5351) -> (-53.3097, 19.5351)
  line L262 (-43.3097, 36.5351) -> (-9.3154, 94.3253)
  line L263 (-64.1903, 14.4649) -> (-93, -35)
  line L264 (-54.1903, 31.4649) -> (-64.1903, 14.4649)
  line L265 (-54.1903, 31.4649) -> (-19.1609, 91.015)
  line L266 (-72.8097, 19.5351) -> (-103, -30)
  line L267 (-62.8097, 36.5351) -> (-72.8097, 19.5351)
  line L268 (-62.8097, 36.5351) -> (-28.8154, 94.3253)
  line L269 (-83.6903, 14.4649) -> (-112.5, -35)
  line L270 (-73.6903, 31.4649) -> (-83.6903, 14.4649)
  line L271 (-73.6903, 31.4649) -> (-38.6609, 91.015)
  line L272 (-92.3097, 19.5351) -> (-122.5, -30)
  line L273 (-82.3097, 36.5351) -> (-92.3097, 19.5351)
  line L274 (-82.3097, 36.5351) -> (-48.3154, 94.3253)
  line L275 (-103.1903, 14.4649) -> (-132, -35)
  line L276 (-93.1903, 31.4649) -> (-103.1903, 14.4649)
  line L277 (-93.1903, 31.4649) -> (-58.1609, 91.015)
  line L278 (-111.8097, 19.5351) -> (-142, -30)
  line L279 (-101.8097, 36.5351) -> (-111.8097, 19.5351)
  line L280 (-101.8097, 36.5351) -> (-67.8154, 94.3253)
  line L281 (-122.6903, 14.4649) -> (-151.5, -35)
  line L282 (-112.6903, 31.4649) -> (-122.6903, 14.4649)
  line L283 (-112.6903, 31.4649) -> (-77.6609, 91.015)
  line L284 (-131.3097, 19.5351) -> (-161.5, -30)
  line L285 (-121.3097, 36.5351) -> (-131.3097, 19.5351)
  line L286 (-121.3097, 36.5351) -> (-87.3154, 94.3253)
  line L287 (-142.1903, 14.4649) -> (-171, -35)
  line L288 (-132.1903, 31.4649) -> (-142.1903, 14.4649)
  line L289 (-132.1903, 31.4649) -> (-97.1609, 91.015)
  line L290 (-150.8097, 19.5351) -> (-181, -30)
  line L291 (-140.8097, 36.5351) -> (-150.8097, 19.5351)
  line L292 (-140.8097, 36.5351) -> (-106.8154, 94.3253)
  line L293 (-161.6903, 14.4649) -> (-190.5, -35)
  line L294 (-151.6903, 31.4649) -> (-161.6903, 14.4649)
  line L295 (-151.6903, 31.4649) -> (-116.6609, 91.015)
  line L296 (-170.3097, 19.5351) -> (-200.5, -30)
  line L297 (-160.3097, 36.5351) -> (-170.3097, 19.5351)
  line L298 (-160.3097, 36.5351) -> (-126.3154, 94.3253)
  line L299 (-181.1903, 14.4649) -> (-210, -35)
  line L300 (-171.1903, 31.4649) -> (-181.1903, 14.4649)
  line L301 (-171.1903, 31.4649) -> (-136.1609, 91.015)
  line L302 (-189.8097, 19.5351) -> (-220, -30)
  line L303 (-179.8097, 36.5351) -> (-189.8097, 19.5351)
  line L304 (-179.8097, 36.5351) -> (-145.8154, 94.3253)
  line L305 (-200.6903, 14.4649) -> (-229.5, -35)
  line L306 (-190.6903, 31.4649) -> (-200.6903, 14.4649)
  line L307 (-190.6903, 31.4649) -> (-155.6609, 91.015)
  line L308 (-209.3097, 19.5351) -> (-239.5, -30)
  line L309 (-199.3097, 36.5351) -> (-209.3097, 19.5351)
  line L310 (-199.3097, 36.5351) -> (-165.3154, 94.3253)
  line L311 (-220.1903, 14.4649) -> (-249, -35)
  line L312 (-210.1903, 31.4649) -> (-220.1903, 14.4649)
  line L313 (-210.1903, 31.4649) -> (-175.1609, 91.015)
  line L314 (-228.8097, 19.5351) -> (-259, -30)
  line L315 (-218.8097, 36.5351) -> (-228.8097, 19.5351)
  line L316 (-218.8097, 36.5351) -> (-184.8154, 94.3253)
  line L317 (-239.6903, 14.4649) -> (-268.5, -35)
  line L318 (-229.6903, 31.4649) -> (-239.6903, 14.4649)
  line L319 (-229.6903, 31.4649) -> (-194.6609, 91.015)
  line L320 (-248.3097, 19.5351) -> (-278.5, -30)
  line L321 (-238.3097, 36.5351) -> (-248.3097, 19.5351)
  line L322 (-238.3097, 36.5351) -> (-204.3154, 94.3253)
  line L323 (-259.1903, 14.4649) -> (-288, -35)
  line L324 (-249.1903, 31.4649) -> (-259.1903, 14.4649)
  line L325 (-249.1903, 31.4649) -> (-214.1609, 91.015)
  line L326 (-267.8097, 19.5351) -> (-298, -30)
  line L327 (-257.8097, 36.5351) -> (-267.8097, 19.5351)
  line L328 (-257.8097, 36.5351) -> (-223.8154, 94.3253)
  line L329 (-278.6903, 14.4649) -> (-307.5, -35)
  line L330 (-268.6903, 31.4649) -> (-278.6903, 14.4649)
  line L331 (-268.6903, 31.4649) -> (-233.6609, 91.015)
  line L332 (-287.3097, 19.5351) -> (-317.5, -30)
  line L333 (-277.3097, 36.5351) -> (-287.3097, 19.5351)
  line L334 (-277.3097, 36.5351) -> (-243.3154, 94.3253)
  line L335 (-298.1903, 14.4649) -> (-327, -35)
  line L336 (-288.1903, 31.4649) -> (-298.1903, 14.4649)
  line L337 (-288.1903, 31.4649) -> (-253.1609, 91.015)
  line L338 (-306.8097, 19.5351) -> (-337, -30)
  line L339 (-296.8097, 36.5351) -> (-306.8097, 19.5351)
  line L340 (-296.8097, 36.5351) -> (-262.8154, 94.3253)
  line L341 (-317.6903, 14.4649) -> (-346.5, -35)
  line L342 (-307.6903, 31.4649) -> (-317.6903, 14.4649)
  line L343 (-307.6903, 31.4649) -> (-272.6609, 91.015)
  line L344 (-326.3097, 19.5351) -> (-356.5, -30)
  line L345 (-316.3097, 36.5351) -> (-326.3097, 19.5351)
  line L346 (-316.3097, 36.5351) -> (-282.3154, 94.3253)
  line L347 (-337.1903, 14.4649) -> (-366, -35)
  line L348 (-327.1903, 31.4649) -> (-337.1903, 14.4649)
  line L349 (-327.1903, 31.4649) -> (-292.1609, 91.015)
  line L350 (-345.8097, 19.5351) -> (-376, -30)
  line L351 (-335.8097, 36.5351) -> (-345.8097, 19.5351)
  line L352 (-335.8097, 36.5351) -> (-301.8154, 94.3253)
  line L353 (-356.6903, 14.4649) -> (-385.5, -35)
  line L354 (-346.6903, 31.4649) -> (-356.6903, 14.4649)
  line L355 (-346.6903, 31.4649) -> (-311.6609, 91.015)
  line L356 (-365.3097, 19.5351) -> (-395.5, -30)
  line L357 (-355.3097, 36.5351) -> (-365.3097, 19.5351)
  line L358 (-355.3097, 36.5351) -> (-321.3154, 94.3253)
  line L359 (70, 85) -> (-388.222, 85)
  line L360 (75, 0) -> (-410, 0)
  line L361 (75, -5) -> (-410, -5)
  line L362 (70, 90) -> (-388.222, 90)
  line L363 (-340.3266, 51) -> (-195.2197, 51)
  line L364 (-340.3266, 56) -> (-195.2197, 56)
  dimension "d314" = 5
  dimension "d315" = 5
  dimension "d322" = 5
  dimension "d324" = 5
  dimension "d328" = -19.5
  dimension "d329" = 0
  dimension "d332" = -19.5
  dimension "d333" = 0
  dimension "d336" = -5
  dimension "d337" = 5
  dimension "d338" = -5
  constraint coincident A21.centre L6.end
  constraint coincident A20.centre L7.end
  constraint parallel L6 L8
  constraint coincident A18.centre L9.start
  constraint coincident A19.centre L8.end
  constraint coincident A22.centre L10.start
  constraint coincident A55.centre L10.end
  constraint coincident A57.centre L11.end
  constraint coincident A17.centre L12.end
  constraint coincident A60.centre L17.start
  constraint coincident A58.centre L17.end
  constraint coincident A54.centre L18.end
  constraint coincident A16.centre L19.end
  constraint coincident A15.centre L22.start
  constraint coincident A52.centre L24.start
  constraint coincident A23.centre L24.end
  constraint coincident A53.centre L25.end
  constraint coincident A59.centre L26.end
  constraint coincident A25.centre L31.start
  constraint coincident A14.centre L31.end
  constraint coincident A24.centre L32.end
  constraint coincident A61.centre L33.end
  constraint coincident A13.centre L36.end
  constraint coincident A63.centre L38.start
  constraint coincident A50.centre L38.end
  constraint coincident A51.centre L39.end
  constraint coincident A62.centre L40.end
  constraint coincident A64.centre L42.end
  constraint coincident A26.centre L46.end
  constraint coincident A12.centre L47.end
  constraint coincident A66.centre L48.end
  constraint coincident A9.centre L49.end
  constraint coincident A47.centre L50.end
  constraint coincident A29.centre L52.start
  constraint coincident A10.centre L52.end
  constraint coincident A28.centre L53.end
  constraint coincident A49.centre L54.end
  constraint coincident A48.centre L57.start
  constraint coincident A11.centre L61.start
  constraint coincident A65.centre L62.end
  constraint coincident A67.centre L63.end
  constraint coincident A46.centre L64.end
  constraint coincident A69.centre L66.start
  constraint coincident A8.centre L66.end
  constraint coincident A30.centre L67.end
  constraint coincident A27.centre L68.end
  constraint coincident A68.centre L70.start
  constraint coincident A31.centre L72.start
  constraint coincident A7.centre L74.start
  constraint coincident A45.centre L74.end
  constraint coincident A32.centre L75.end
  constraint coincident A6.centre L76.start
  constraint coincident A44.centre L76.end
  constraint coincident A43.centre L77.end
  constraint coincident A5.centre L79.end
  constraint coincident A70.centre L81.start
  constraint coincident A71.centre L81.end
  constraint coincident A33.centre L82.start
  constraint coincident A34.centre L83.end
  constraint coincident A72.centre L84.end
  constraint coincident A41.centre L85.end
  constraint coincident A4.centre L87.end
  constraint coincident A42.centre L89.start
  constraint coincident A35.centre L89.end
  constraint coincident A3.centre L90.end
  constraint coincident A74.centre L91.end
  constraint coincident A36.centre L92.end
  constraint coincident A2.centre L93.end
  constraint coincident A73.centre L94.end
  constraint coincident A38.centre L95.start
  constraint coincident A75.centre L95.end
  constraint coincident A37.centre L96.end
  constraint coincident A1.centre L97.end
  constraint coincident A0.centre L98.end
  constraint coincident A39.centre L99.start
  constraint coincident A40.centre L101.start
  constraint coincident L5.start A81.centre
  constraint coincident L13.end L14.start
  constraint coincident L15.end L16.start
  constraint coincident L14.end L15.start
  constraint coincident L21.end A80.centre
  constraint coincident L20.end L21.start
  constraint coincident L28.end L29.start
  constraint coincident L29.end L30.start
  constraint coincident L27.end L28.start
  constraint coincident L35.end A94.centre
  constraint coincident L44.end A78.centre
  constraint coincident L45.start A85.centre
  constraint coincident L45.end L46.start
  constraint coincident L55.end L56.start
  constraint coincident L56.end A77.centre
  constraint coincident L59.start L60.end
  constraint coincident L59.end L61.end
  constraint coincident L60.start L65.start
  constraint coincident L41.end L42.start
  constraint coincident L69.end L71.start
  constraint coincident L96 A75.centre
  constraint horizontal L109
  constraint coincident L71 A68.centre
  constraint parallel L120 L121
  constraint coincident A56.centre L128.start
  constraint parallel L108 L130
  constraint horizontal L131
  constraint parallel L108 L132
  constraint parallel L130 L133
  constraint parallel L132 L134
  constraint coincident L95 L131.start
  constraint parallel L132 L135
  constraint parallel L140 L141
  constraint parallel L139 L142
  constraint parallel L144 L145
  constraint parallel L143 L146
  constraint parallel L139 L149
  constraint horizontal L359
  constraint horizontal L360
  constraint midpoint L121 L363.end
  constraint parallel L121 L363
  measures "d314" distance of L108 L132
  measures "d315" distance of L108 L130
extrude "Extrude15" cut sketch "Sketch2" against normal blind 2.2 contours L344 L347 L360 L361 | L132 L133 L134 L138 L244 L347 L348 L350 L351 L360 | L135 L137 L341 L344 L360 L361 | L132 L344 L347 L360 | L338 L341 L360 L361 | L132 L135 L344 L360 | L130 L132 L133 L344 L347 L348 | L132 L133 L134 L138 L347 L348 | L241 L244 L348 L349 L351 L352 | L244 L338 L360 L361 | L130 L136 L137 L244 L341 L344 L360 | L244 L338 L341 L360 | L130 L132 L135 L136 L137 L344 L360 | L135 L137 L360 | L241 L244 L344 L345 L348 L349 | L130 L133 L244 L344 L348 | L241 L244 L338 L341 L342 | L241 L244 L341 L342 L344 L345 | L239 L241 L349 L352 | L241 L244 L335 L338 L360 | L236 L239 L349 L352 L363 | L236 L239 L335 L336 L338 L339 | L236 L239 L338 L339 L342 L343 | L236 L239 L342 L343 L345 L346 | L236 L239 L332 L335 L336 | L234 L236 L343 L346 | L236 L239 L329 L332 L360 | L234 L236 L336 L339 | L234 L236 L339 L343 | L231 L234 L343 L346 L363 | L234 L236 L329 L332 | L234 L236 L332 L336 | L231 L234 L336 L337 L339 L340 | L231 L234 L339 L340 L343 | L231 L234 L329 L330 L332 L333 | L231 L234 L332 L333 L336 L337 | L229 L231 L340 L343 L363 | L231 L343 L363 | L231 L343 L363 L364 | L229 L231 L337 L340 | L229 L343 L363 L364 | L231 L323 L360 L361 | L231 L234 L323 L326 L360 | L226 L229 L337 L340 L363 | L229 L340 L363 | L229 L340 L363 L364 | L231 L323 L360 | L231 L320 L360 L361 | L229 L231 L323 L326 | L226 L229 L330 L331 L333 L334 | L229 L320 L360 L361 | L229 L231 L320 L323 L360 | L226 L229 L323 L324 L326 L327 | L226 L229 L326 L327 L330 L331 | L229 L320 L360 | L226 L229 L320 L323 L324 | L224 L226 L331 L334 | L226 L229 L317 L320 L360 | L224 L226 L324 L327 | L224 L226 L327 L331 | L221 L224 L331 L334 L363 | L221 L224 L324 L325 L327 L328 | L221 L224 L327 L328 L331 | L221 L334 L363 L364 | L221 L224 L317 L318 L320 L321 | L219 L221 L328 L331 L363 | L221 L331 L363 L364 | L221 L224 L314 L317 L318 | L219 L221 L325 L328 | L219 L331 L363 L364 | L221 L311 L360 L361 | L221 L224 L311 L314 L360 | L219 L221 L318 L321 | L216 L219 L325 L328 L363 | L219 L328 L363 L364 | L221 L308 L360 L361 | L219 L221 L311 L314 | L219 L221 L314 L318 | L216 L219 L318 L319 L321 L322 | L216 L328 L363 L364 | L219 L308 L360 L361 | L219 L221 L308 L311 L360 | L216 L219 L311 L312 L314 L315 | L216 L219 L314 L315 L318 L319 | L216 L219 L308 L311 L312 | L214 L216 L319 L322 | L216 L219 L305 L308 L360 | L214 L216 L312 L315 | L214 L216 L315 L319 | L211 L214 L319 L322 L363 | L211 L214 L312 L313 L315 L316 | L211 L214 L315 L316 L319 | L211 L322 L363 L364 | L211 L214 L305 L306 L308 L309 | L211 L214 L302 L305 L306 | L211 L214 L299 L302 L360 | L209 L211 L306 L309 | L206 L209 L313 L316 L363 | L209 L211 L299 L302 | L209 L211 L302 L306 | L206 L209 L306 L307 L309 L310 | L206 L209 L309 L310 L313 | L206 L316 L363 L364 | L206 L209 L299 L300 L302 L303 | L206 L209 L302 L303 L306 L307 | L204 L206 L310 L313 | L206 L313 L363 | L206 L316 L364 | L206 L313 L363 L364 | L204 L206 L307 L310 | L203 L204 L206 L313 L316 L364 | L200 L201 L203 L204 L313 L316 | L206 L209 L293 L296 L360 | L201 L204 L307 L310 | L201 L204 L310 L313 | L204 L206 L293 L296 | L201 L204 L300 L301 L303 L304 | L201 L204 L293 L294 L296 L297 | L201 L204 L296 L297 L300 L301 | L195 L196 L198 L199 L307 L310 | L192 L193 L195 L196 L307 L310 | L190 L192 L193 L307 L310 L359 | L199 L201 L301 L304 | L196 L199 L304 L307 | L201 L204 L287 L290 L360 | L196 L199 L301 L304 | L193 L196 L304 L307 | L190 L193 L304 L307 | L199 L201 L287 L290 | L196 L199 L294 L295 L297 L298 | L193 L194 L196 L301 L304 | L190 L191 L193 L194 L301 L304 | L185 L187 L188 L301 L304 L359 | L196 L199 L287 L288 L290 L291 | L196 L199 L290 L291 L294 L295 | L194 L196 L295 L298 | L185 L188 L298 L301 | L196 L281 L360 L361 | L196 L199 L281 L284 L360 | L194 L196 L288 L291 | L194 L196 L291 L295 | L191 L194 L295 L298 | L188 L189 L191 L295 L298 | L185 L186 L188 L189 L295 L298 | L180 L182 L183 L295 L298 L359 | L196 L278 L360 L361 | L194 L196 L281 L284 | L191 L194 L288 L289 L291 L292 | L191 L194 L291 L292 L295 | L194 L278 L360 L361 | L194 L196 L278 L281 L360 | L191 L194 L281 L282 L284 L285 | L180 L183 L292 L295 | L191 L194 L278 L281 L282 | L186 L189 L289 L292 | L183 L184 L186 L289 L292 | L180 L181 L183 L184 L289 L292 | L175 L177 L178 L289 L292 L359 | L191 L194 L275 L278 L360 | L189 L191 L282 L285 | L186 L189 L285 L286 L289 | L186 L189 L282 L283 L285 L286 | L175 L178 L286 L289 | L186 L189 L275 L276 L278 L279 | L181 L184 L283 L286 | L178 L179 L181 L283 L286 | L175 L176 L178 L179 L283 L286 | L170 L172 L173 L283 L286 L359 | L186 L189 L272 L275 L276 | L184 L186 L276 L279 | L181 L184 L279 L280 L283 | L179 L181 L280 L283 | L186 L189 L269 L272 L360 | L181 L184 L276 L277 L279 L280 | L179 L181 L277 L280 | L176 L179 L280 L283 | L170 L173 L280 L283 | L277 L280 L359 L362 | L176 L179 L277 L280 | L170 L171 L173 L174 L277 L280 | L165 L167 L168 L277 L280 L359 | L162 L277 L359 L362 | L181 L184 L269 L270 L272 L273 | L179 L181 L270 L273 | L162 L165 L274 L277 L359 | L162 L274 L359 L362 | L181 L184 L266 L269 L270 | L179 L181 L266 L270 | L176 L179 L270 L271 L273 L274 | L174 L176 L271 L274 | L171 L174 L274 L277 | L165 L168 L274 L277 | L181 L184 L263 L266 L360 | L179 L181 L263 L266 | L176 L179 L266 L267 L270 L271 | L171 L174 L271 L274 | L165 L166 L168 L169 L271 L274 | L162 L163 L165 L166 L271 L274 | L160 L162 L163 L271 L274 L359 | L176 L179 L263 L264 L266 L267 | L171 L174 L264 L265 L267 L268 | L169 L171 L265 L268 | L166 L169 L268 L271 | L176 L179 L257 L260 L360 | L174 L176 L257 L260 | L171 L174 L260 L261 L264 L265 | L166 L169 L265 L268 | L160 L161 L163 L164 L265 L268 | L157 L158 L160 L161 L265 L268 | L155 L157 L158 L265 L268 L359 | L171 L174 L257 L258 L260 L261 | L166 L169 L258 L259 L261 L262 | L164 L166 L259 L262 | L161 L164 L262 L265 | L171 L174 L251 L254 L360 | L169 L171 L251 L254 | L166 L169 L254 L255 L258 L259 | L164 L166 L255 L259 | L161 L164 L259 L262 | L155 L156 L158 L159 L259 L262 | L152 L153 L155 L156 L259 L262 | L150 L152 L153 L259 L262 L359 | L166 L169 L251 L252 L254 L255 | L164 L166 L252 L255 | L161 L164 L255 L256 L259 | L161 L164 L252 L253 L255 L256 | L156 L159 L256 L259 | L153 L156 L256 L259 | L150 L153 L256 L259 | L166 L169 L245 L248 L360 | L164 L166 L245 L248 | L156 L159 L253 L256 | L153 L154 L156 L253 L256 | L150 L151 L153 L154 L253 L256 | L139 L140 L149 L253 L256 L359 | L161 L164 L245 L246 L248 L249 | L159 L161 L246 L249 | L156 L159 L249 L250 L253 | L156 L159 L246 L247 L249 L250 | L139 L140 L250 L253 | L147 L148 L161 L164 L360 | L147 L148 L159 L161 | L151 L154 L247 L250 | L139 L142 L151 L247 L250 | L139 L140 L141 L142 L247 L250 | L143 L144 L147 L148 L156 L159 | L148 L159 L161 L360 | L143 L144 L154 L156 | L143 L146 L151 L154 L247 | L148 L161 L360 L361 | L144 L148 L156 L159 L360 | L159 L161 L360 L361 | L143 L144 L145 L146 L151 L154 bodies 1
ref_plane "WorkPlane1" through (35.5, 169, 43) normal (1, 0, 0) x (0, 1, 0)
box "BoxPrimitive1" add length 10 width 144 height 62 placed x (0, 0, -1) y (0, 1, 0) z (1, 0, 0) at (0, 193.4134, 132.5024) separate body makes body 2
move_body "Move1" bodies 2 to x (1, 0, 0) y (0, 0.987688, -0.156434) z (0, 0.156434, 0.987688) at (5, -30.4825, -5.6254)
combine "Combine2" operation cut target body 1 tool bodies 2 keep tools
mirror "Mirror1" about plane through (35.5, 169, 43) normal (1, 0, 0) of bodies 1 makes body 3